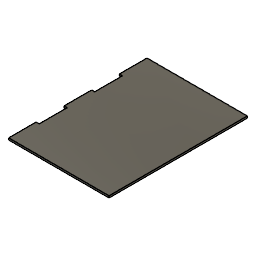
Expandable Notebook (Autodesk Fusion 360 design; units mm, degrees)
Autodesk Fusion 360 part; units mm, degrees
sketch "Sketch1" plane through (0, 0, 0) normal (0, 0, 1) x (1, 0, 0)
  line L0 (0, 0) -> (-148.5, 0)
  line L1 (-148.5, 0) -> (-148.5, 210)
  line L2 (-148.5, 210) -> (0, 210)
  line L3 (0, 210) -> (0, 0)
  line L4 (0, 0) -> (7.0711, -7.0711)
  line L5 (0, 0) -> (10, 0) construction
  line L6 (-148.5, 210) -> (-155.5711, 217.0711)
  line L7 (-148.5, 210) -> (-138.5, 210) construction
  line L8 (-155.5711, 217.0711) -> (7.0711, 217.0711)
  line L9 (7.0711, 217.0711) -> (7.0711, -7.0711)
  line L10 (7.0711, -7.0711) -> (-155.5711, -7.0711)
  line L11 (-155.5711, -7.0711) -> (-155.5711, 217.0711)
  dimension "d1" = 148.5
  dimension "d2" = 210
  dimension "d3" = 10
  dimension "d4" = 45
  dimension "d5" = 135
  dimension "d6" = 10
  constraint horizontal L0
  constraint vertical L1
  constraint horizontal L2
  constraint vertical L3
  constraint coincident L0.start L3.end
  constraint horizontal L5
  constraint horizontal L7
  constraint horizontal L8
  constraint vertical L9
  constraint horizontal L10
  constraint vertical L11
  measures "d1" distance of L0.start L0.end
  measures "d2" distance of L0.start L2.end
  measures "d3" distance of L0.start L4.end
  measures "d4" angle of L4 L5
  measures "d5" angle of L6 L7
  measures "d6" distance of L1.end L6.end
extrude "Extrude1" add sketch "Sketch1" along normal blind 3
sketch "Sketch2" plane through (0, 0, 3) normal (0, 0, 1) x (-1, 0, 0)
  line L0 (155.5711, 7.0711) -> (-7.0711, 7.0711)
  line L1 (-7.0711, 7.0711) -> (-7.0711, -217.0711)
  line L2 (-7.0711, -217.0711) -> (155.5711, -217.0711)
  line L3 (155.5711, -217.0711) -> (155.5711, 7.0711)
  line L4 (155.5711, 7.0711) -> (145.5711, 7.0711)
  line L5 (145.5711, 7.0711) -> (145.5711, -217.0709)
  line L6 (145.5711, -217.0709) -> (155.5711, -217.0709)
  line L7 (155.5711, -217.0709) -> (155.5711, 7.0711)
  line L8 (155.5711, -217.0711) -> (150.5711, -217.0711)
  line L9 (150.5711, -217.0711) -> (150.5711, -172.2427)
  line L10 (150.5711, -172.2427) -> (155.5711, -172.2427)
  line L11 (155.5711, -172.2427) -> (155.5711, -217.0711)
  line L12 (150.5711, -172.2427) -> (155.5711, -172.2427)
  line L13 (155.5711, -172.2427) -> (155.5711, -127.4143)
  line L14 (155.5711, -127.4143) -> (150.5711, -127.4143)
  line L15 (150.5711, -127.4143) -> (150.5711, -172.2427)
  line L16 (150.5711, -127.4143) -> (155.5711, -127.4143)
  line L17 (155.5711, -127.4143) -> (155.5711, -82.5859)
  line L18 (155.5711, -82.5859) -> (150.5711, -82.5859)
  line L19 (150.5711, -82.5859) -> (150.5711, -127.4143)
  line L20 (150.5711, -82.5859) -> (155.5711, -82.5859)
  line L21 (155.5711, -82.5859) -> (155.5711, -37.7575)
  line L22 (155.5711, -37.7575) -> (150.5711, -37.7575)
  line L23 (150.5711, -37.7575) -> (150.5711, -82.5859)
  line L24 (150.5711, -37.7575) -> (155.5711, -37.7575)
  line L25 (155.5711, -37.7575) -> (155.5711, 7.0711)
  line L26 (155.5711, 7.0711) -> (150.5711, 7.0711)
  line L27 (150.5711, 7.0711) -> (150.5711, -37.7575)
  dimension "d9" = 10
  dimension "d10" = 224.142
  dimension "d11" = 44.8284
  dimension "d12" = 44.8284
  dimension "d13" = 44.8284
  dimension "d14" = 44.8284
  constraint horizontal L4
  constraint vertical L5
  constraint horizontal L6
  constraint vertical L7
  constraint coincident L0.start L3.end
  constraint horizontal L8
  constraint vertical L9
  constraint horizontal L10
  constraint vertical L11
  constraint coincident L2.end L3.start
  constraint horizontal L12
  constraint vertical L13
  constraint horizontal L14
  constraint vertical L15
  constraint horizontal L16
  constraint vertical L17
  constraint horizontal L18
  constraint vertical L19
  constraint coincident L7 L17.end
  constraint horizontal L20
  constraint vertical L21
  constraint horizontal L22
  constraint vertical L23
  constraint coincident L7 L21.end
  constraint horizontal L24
  constraint vertical L25
  constraint horizontal L26
  constraint vertical L27
  measures "d9" distance of L0.start L4.end
  measures "d10" distance of L0.start L6.end
  measures "d11" distance of L2.end L10.end
  measures "d12" distance of L9.end L14.end
  measures "d13" distance of L14.end L18.end
  measures "d14" distance of L18.end L22.end
extrude "Extrude2" cut sketch "Sketch2" against normal blind 160 contours L3 L7 L18 L20 L21 L22 L23 L24 | L3 L7 L10 L12 L13 L14 L15 L16
